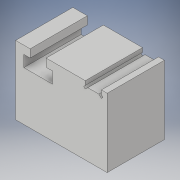
# Autodesk Inventor part: PiesaSuportCanale
Saved by Autodesk Inventor 2019 (Build 230136000, 136)
## iProperties
Created: 2019-03-11
Part Number: PiesaSuportCanale
Material: Generic
Document SubType Name: Modeling
Designer: forev
Density: 1 g/cm^3
Appearance: Default
Author: forev
Autodesk Inventor part; units mm, degrees
ref_plane "YZ Plane" through (0, 0, 0) normal (1, 0, 0) x (0, 1, 0)
ref_plane "XZ Plane" through (0, 0, 0) normal (0, 1, 0) x (-1, 0, 0)
ref_plane "XY Plane" through (0, 0, 0) normal (0, 0, 1) x (1, 0, 0)
sketch "Sketch1" plane through (0, 0, 0) normal (0, 0, 1) x (1, 0, 0)
  line L0 (-42.7621, 33.3504) -> (37.2379, 33.3504)
  line L1 (37.2379, 33.3504) -> (37.2379, -26.6496)
  line L2 (37.2379, -26.6496) -> (-42.7621, -26.6496)
  line L3 (-42.7621, -26.6496) -> (-42.7621, 33.3504)
  point P0 (0, 0)
  dimension "d0" = 80
  dimension "d1" = 60
  constraints: 8 end point, 2 parallel, 1 horizontal, 1 perpendicular
  measures "d0" distance of L0.start L0.end
  measures "d1" distance of L0.end L1.end
extrude "Extrusion1" add sketch "Sketch1" along normal blind 50
sketch "Sketch2" plane through (0, 0, 50) normal (0, 0, 1) x (1, 0, 0)
  line L0 (-30.0743, 35.3951) -> (-16.0743, 35.3951)
  line L1 (-16.0743, 35.3951) -> (-16.0743, 26.3951)
  line L2 (-16.0743, 26.3951) -> (-10.5743, 26.3951)
  line L3 (-10.5743, 26.3951) -> (-10.5743, 16.3951)
  line L4 (-10.5743, 16.3951) -> (-35.5743, 16.3951)
  line L5 (-35.5743, 16.3951) -> (-35.5743, 26.3951)
  line L6 (-35.5743, 26.3951) -> (-30.0743, 26.3951)
  line L7 (-30.0743, 26.3951) -> (-30.0743, 35.3951)
  point P0 (0, 0)
  point P1 (-23.0743, 35.3951)
  dimension "d4" = 14
  dimension "d5" = 25
  dimension "d6" = 10
  dimension "d7" = 9
  dimension "d8" = 7
  dimension "d9" = 12.5
  constraints: 16 end point, 6 perpendicular, 2 point on line, 1 horizontal, 1 midpoint
  measures "d4" distance of L0.start L0.end
  measures "d5" distance of L3.end L4.end
  measures "d6" distance of L4.end L5.end
  measures "d7" distance of L6.end L0.start
  measures "d8" distance of L0.start point (-23.074, 35.395)
  measures "d9" distance from line of L5 point (-23.074, 35.395)
extrude "Extrusion2" cut sketch "Sketch2" against normal blind 50
sketch "Sketch3" plane through (0, 0, 50) normal (0, 0, 1) x (1, 0, 0)
  line L0 (25.1509, 34.1359) -> (32.1509, 34.1359)
  line L1 (32.1509, 34.1359) -> (32.1509, 29.8137)
  line L2 (32.1509, 29.8137) -> (33.5651, 28.3995)
  line L3 (33.5651, 28.3995) -> (32.1509, 26.9853)
  line L4 (32.1509, 26.9853) -> (30.0002, 29.1359)
  line L5 (30.0002, 29.1359) -> (25.1509, 29.1359)
  line L6 (25.1509, 34.1359) -> (25.1509, 29.1359) construction
  line L7 (25.1509, 34.1359) -> (18.1509, 34.1359)
  line L8 (18.1509, 34.1359) -> (18.1509, 29.8137)
  line L9 (18.1509, 29.8137) -> (16.7366, 28.3995)
  line L10 (16.7366, 28.3995) -> (18.1509, 26.9853)
  line L11 (18.1509, 26.9853) -> (20.3015, 29.1359)
  line L12 (20.3015, 29.1359) -> (25.1509, 29.1359)
  point P0 (0, 0)
  dimension "d12" = 7
  dimension "d13" = 5
  dimension "d14" = 2
  dimension "d15" = 2
  dimension "d16" = 135
  dimension "d17" = 4.3222
  constraints: 26 end point, 5 symmetric about line, 3 coincident, 3 perpendicular, 2 point on line, 1 horizontal, 1 parallel, 1 vertical
  measures "d12" distance of L0.start L0.end
  measures "d13" distance between parallel lines of L5 L0
  measures "d14" distance of L1.end L2.end
  measures "d15" distance of L2.end L3.end
  measures "d16" angle of L4 L5
  measures "d17" distance of L0.end L1.end
extrude "Extrusion3" cut sketch "Sketch3" against normal blind 50
body "Solid1"
